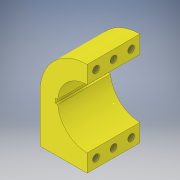
# Autodesk Inventor part: gripperBracketA
Saved by Autodesk Inventor 2018.2 (Build 222227000, 227)
## iProperties
Created: 2018-02-13
Part Number: gripperBracketA
Material: Aluminum 6061
Document SubType Name: Modeling
Designer: steele
Density: 2.7 g/cm^3
Appearance: Canary
Author: steele
Autodesk Inventor part; units mm, degrees
ref_plane "YZ Plane" through (0, 0, 0) normal (1, 0, 0) x (0, 1, 0)
ref_plane "XZ Plane" through (0, 0, 0) normal (0, 1, 0) x (-1, 0, 0)
ref_plane "XY Plane" through (0, 0, 0) normal (0, 0, 1) x (1, 0, 0)
sketch "Sketch1" plane through (0, 0, 0) normal (0, 0, 1) x (1, 0, 0)
  arc A0 (-21.2132, -1.5875) -> (-21.2132, 1.5875) centre (0, 0) ccw
  arc A1 (0, 33.9725) -> (-33.9725, 0) centre (0, 0) ccw
  line L0 (0, -33.9725) -> (-33.9725, -33.9725)
  line L1 (-33.9725, 0) -> (-33.9725, -33.9725)
  line L2 (0, 33.9725) -> (33.9725, 33.9725)
  line L3 (0, -33.9725) -> (33.9725, -33.9725)
  line L4 (33.9725, 0) -> (33.9725, -33.9725)
  line L5 (33.9725, 0) -> (33.9725, 33.9725)
  line L6 (0, 0) -> (-21.2655, 0) construction
  line L7 (-21.2132, 1.5875) -> (-22.8007, 1.5875)
  line L8 (-22.8007, 1.5875) -> (-22.8007, -1.5875)
  line L9 (-22.8007, -1.5875) -> (-21.2132, -1.5875)
  dimension "d0" = 42.545
  dimension "d1" = 67.945
  dimension "d29" = 1.5875
  dimension "d30" = 1.5875
  dimension "d31" = 1.5875
  constraints: 20 end point, 5 horizontal, 5 perpendicular, 5 tangent, 4 point on circle, 2 centre point, 2 coincident
  measures "d0" diameter of A0
  measures "d1" diameter of A1
  measures "d29" distance of L7.start L7.end
  measures "d30" distance from line of L7.end L6
  measures "d31" distance between parallel lines of L6 L9
extrude "Extrusion1" add sketch "Sketch1" along normal mid plane 38.1
sketch "Sketch3" plane through (33.9725, -33.9725, 19.05) normal (1, 0, 0) x (0, 0, -1)
  line L0 (0, 67.945) -> (38.1, 67.945) construction
  line L1 (19.05, 67.945) -> (19.05, 0) construction
  line L2 (0, 0) -> (38.1, 0) construction
  point P0 (19.05, 33.9725)
  point P1 (19.05, 61.595)
  point P2 (19.05, 6.35)
  dimension "d13" = 6.35
  dimension "d14" = 6.35
  constraints: 2 end point, 2 midpoint, 2 point on line
  measures "d13" distance from line of point (19.05, 61.595) L0
  measures "d14" distance from line of point (19.05, 6.35) L2
split "Split1" plane through (0, 0, 0) removes the side toward (1, 0, 0)
sketch "Sketch4" plane through (0, 21.2725, -19.05) normal (1, 0, 0) x (0, 0, -1)
  point P0 (-19.05, -21.2725)
hole "Hole3" at (33.9725, 27.6225, 0) at (33.9725, -27.6225, 0) direction (-1, 0, 0) diameter 4.9784 depth 46.355 tip angle 118 thread size "1/4-20 UNC" class "2B" standard "ANSI Unified Screw Threads"
sketch "Sketch5" plane through (-33.9725, -33.9725, 19.05) normal (-1, 0, 0) x (0, 0, 1)
  line L0 (0, 0) -> (-38.1, 0) construction
  line L1 (-31.75, 0) -> (-31.75, 33.9725) construction
  line L2 (-6.35, 0) -> (-6.35, 33.9725) construction
  line L3 (0, 33.9725) -> (-38.1, 33.9725) construction
  line L4 (-38.1, 0) -> (-38.1, 33.9725) construction
  line L5 (0, 33.9725) -> (0, 0) construction
  line L6 (-19.05, 33.9725) -> (-19.05, 0) construction
  point P0 (-31.75, 10.16)
  point P1 (-6.35, 10.16)
  point P2 (-19.05, 10.16)
  dimension "d32" = 6.35
  dimension "d33" = 6.35
  dimension "d34" = 10.16
  dimension "d35" = 10.16
  constraints: 6 end point, 6 point on line, 2 vertical, 1 midpoint
  measures "d32" distance between parallel lines of L1 L4
  measures "d33" distance between parallel lines of L5 L2
  measures "d34" distance from line of point (-31.75, 10.16) L0
  measures "d35" distance from line of L0 point (-6.35, 10.16)
sketch "Sketch6" plane through (0, -33.9725, 19.05) normal (1, 0, 0) x (0, 0, -1)
  line L0 (0, 67.945) -> (38.1, 67.945) construction
  line L1 (6.35, 67.945) -> (6.35, 0) construction
  line L2 (0, 0) -> (38.1, 0) construction
  line L3 (31.75, 67.945) -> (31.75, 0) construction
  line L4 (0, 0) -> (0, 12.7) construction
  line L5 (38.1, 12.7) -> (38.1, 0) construction
  point P0 (19.05, 33.9725)
  point P1 (6.35, 6.35)
  point P2 (6.35, 61.595)
  point P3 (31.75, 61.595)
  point P4 (31.75, 6.35)
  dimension "d36" = 6.35
  dimension "d37" = 6.35
  dimension "d38" = 6.35
  dimension "d39" = 6.35
  constraints: 6 point on line, 4 end point, 2 vertical
  measures "d36" distance between parallel lines of L1 L4
  measures "d37" distance between parallel lines of L3 L5
  measures "d38" distance from line of point (6.35, 61.595) L0
  measures "d39" distance from line of point (31.75, 61.595) L0
hole "Hole4" at (-33.9725, -23.8125, -12.7) at (-33.9725, -23.8125, 0) at (-33.9725, -23.8125, 12.7) direction (1, 0, 0) diameter 4.9784 depth 25.4 tip angle 118 thread size "1/4-20 UNC" class "2B" standard "ANSI Unified Screw Threads"
hole "Hole5" at (0, 27.6225, 12.7) at (0, 27.6225, -12.7) at (0, -27.6225, -12.7) at (0, -27.6225, 12.7) direction (-1, 0, 0) diameter 4.9784 depth 9.525 tip angle 118 thread size "1/4-20 UNC" class "2B" standard "ANSI Unified Screw Threads"
equation "\"d0\" = pipeDiameter"
equation "\"d1\" = pipeDiameter + 2 * outerRadius"
equation "\"d2\" = width"
equation "\"pipeDiameter\" = 42.545"
equation "\"outerRadius\" = 12.7"
equation "\"width\" = 38.1"
body "Solid1"
